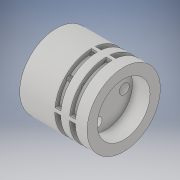
# Autodesk Inventor part: felga
Saved by Autodesk Inventor 2019 (Build 230136000, 136)
## iProperties
Created: 2019-09-09
Part Number: felga
Material: Generic
Document SubType Name: Modeling
Designer: Michal
Density: 1 g/cm^3
Appearance: Default
Author: Michal
Autodesk Inventor part; units mm, degrees
ref_plane "YZ Plane" through (0, 0, 0) normal (1, 0, 0) x (0, 1, 0)
ref_plane "XZ Plane" through (0, 0, 0) normal (0, 1, 0) x (-1, 0, 0)
ref_plane "XY Plane" through (0, 0, 0) normal (0, 0, 1) x (1, 0, 0)
sketch "Sketch1" plane through (0, 0, 0) normal (1, 0, 0) x (0, 1, 0)
  circle A0 centre (0, 0) radius 12.5
  circle A1 centre (0, 0) radius 11
  dimension "d0" = 25
  dimension "d1" = 22
  constraints: 2 centre point, 2 coincident
  measures "d0" diameter of A0
  measures "d1" diameter of A1
extrude "Extrusion1" add sketch "Sketch1" along normal blind 6.5
sketch "Sketch2" plane through (6.5, 0, 0) normal (1, 0, 0) x (0, 0, -1)
  circle A0 centre (0, 0) radius 9
  circle A1 centre (0, 0) radius 12.5
  dimension "d4" = 18
  constraints: 2 centre point, 2 coincident
  measures "d4" diameter of A0
extrude "Extrusion2" add sketch "Sketch2" along normal blind 5.5
sketch "Sketch3" plane through (12, 0, 0) normal (1, 0, 0) x (0, 0, -1)
  circle A0 centre (0, 0) radius 11
  dimension "d55" = 22
  constraints: 1 centre point, 1 coincident
  measures "d55" diameter of A0
extrude "Extrusion3" add sketch "Sketch3" along normal blind 2
sketch "Sketch4" plane through (14, 0, 0) normal (1, 0, 0) x (0, 0, -1)
  circle A0 centre (0, 0) radius 12.5
  constraints: 1 centre point, 1 coincident
extrude "Extrusion4" add sketch "Sketch4" along normal blind 3
sketch "Sketch5" plane through (17, 0, 0) normal (1, 0, 0) x (0, 0, -1)
  circle A0 centre (0, 0) radius 9
  circle A1 centre (0, 0) radius 11
  dimension "d54" = 22
  constraints: 2 centre point, 2 coincident
  measures "d54" diameter of A1
extrude "Extrusion5" add sketch "Sketch5" along normal blind 2
sketch "Sketch7" plane through (17, 0, 0) normal (1, 0, 0) x (0, 0, -1)
  line L0 (0, 0) -> (6.2, 0)
  line L1 (0, 0) -> (-3.1, 5.3694)
  line L2 (0, 0) -> (6.2, 0) construction
  line L3 (0, 0) -> (-3.1, -5.3694)
  line L4 (0, 0) -> (6.2, 0) construction
  dimension "d15" = 6.2
  dimension "d16" = 6.2
  dimension "d17" = 120
  dimension "d18" = 6.2
  dimension "d19" = 120
  constraints: 10 end point, 3 horizontal, 2 equal length
  measures "d15" distance of L0.start L0.end
  measures "d16" distance of L0.start L1.end
  measures "d17" angle of L2 L1
  measures "d18" distance of L0.start L3.end
  measures "d19" angle of L3 L4
hole "Hole1" at (17, 5.3694, 3.1) at (17, 0, -6.2) at (17, -5.3694, 3.1) direction (-1, 0, 0) diameter 3.4 end through all clearance for "Countersunk Flat Head Screw ISO 2009/7046" size "M3" standard "ISO"
sketch "Sketch8" plane through (12, 0, 0) normal (1, 0, 0) x (0, 0, -1)
  circle A0 centre (0, 0) radius 9
  circle A1 centre (0, 0) radius 9 projected
  circle A2 centre (0, 0) radius 12.5
  line L0 (-9, 0) -> (-12.5, 0)
  line L1 (-8.9507, 0.9408) -> (-12.4315, 1.3066)
  line L2 (-0.9408, -8.9507) -> (-1.3066, -12.4315)
  circle A3 centre (0, 0) radius 12.5 projected
  line L3 (0, -12.5) -> (0, -9)
  line L4 (9, 0) -> (12.5, 0)
  line L5 (0.9408, 8.9507) -> (1.3066, 12.4315)
  line L6 (0, 12.5) -> (0, 9)
  line L7 (-0.2849, 0.0299) -> (8.8591, 0.0299) construction
  line L8 (8.9507, -0.9408) -> (12.4315, -1.3066)
  constraints: 18 end point, 3 horizontal, 3 point on circle, 2 centre point, 2 vertical, 1 coincident, 1 point on line, 15 other
extrude "Extrusion7" add sketch "Sketch8" along normal blind 7 contours L4 A2 L8 A0 | A0 L6 A2 L5 | L3 A2 L2 A0 | A0 L0 A2 L1
sketch "Sketch10" plane through (17, 0, 0) normal (1, 0, 0) x (0, 0, -1)
  circle A0 centre (0, 0) radius 11
  circle A1 centre (0, 11) radius 0.75
  arc A2 (-11, 0) -> (-1.1498, -10.9397) centre (0, 0) ccw projected
  circle A3 centre (-11, 0) radius 0.75
  line L0 (0, -11) -> (0, -12.5) projected
  circle A4 centre (0, -11) radius 0.75
  circle A5 centre (11, 0) radius 0.75
  line L1 (0, 0) -> (10.9982, 0) construction
  line L2 (0, 0) -> (7.7782, 7.7782)
  line L3 (0, 0) -> (11, 0) construction
  circle A6 centre (7.7782, 7.7782) radius 0.75
  line L4 (0, 0) -> (-7.7782, 7.7782)
  line L5 (0, 0) -> (-7.7782, -7.7782)
  line L6 (0, 0) -> (7.7782, -7.7782)
  circle A7 centre (-7.7782, -7.7782) radius 0.75
  circle A8 centre (7.7782, -7.7782) radius 0.75
  circle A9 centre (-7.7782, 7.7782) radius 0.75
  dimension "d60" = 1.5
  dimension "d61" = 1.5
  dimension "d62" = 1.5
  dimension "d63" = 1.5
  dimension "d66" = 11
  dimension "d67" = 45
  dimension "d68" = 1.5
  dimension "d69" = 11
  dimension "d70" = 11
  dimension "d71" = 11
  dimension "d72" = 1.5
  dimension "d73" = 1.5
  dimension "d74" = 1.5
  constraints: 12 end point, 9 centre point, 5 coincident, 2 horizontal, 2 point on circle, 1 equal length
  measures "d60" diameter of A1
  measures "d61" diameter of A3
  measures "d62" diameter of A4
  measures "d63" diameter of A5
  measures "d66" distance of L1.start L2.end
  measures "d67" angle of L3 L2
  measures "d68" diameter of A6
  measures "d69" distance of L1.start L4.end
  measures "d70" distance of L1.start L5.end
  measures "d71" distance of L1.start L6.end
  measures "d72" diameter of A7
  measures "d73" diameter of A8
  measures "d74" diameter of A9
extrude "Extrusion8" cut sketch "Sketch10" against normal blind 7 contours A0 A5 | A0 A5 | A6 L2 A0 | A0 A6 | A8 A0 | A0 L6 A8 | L2 A6 A0 | A0 A8 L6 | A1 A0 | A0 A1 | A9 A0 L4 | L4 A0 A9 | A7 A0 L5 | L5 A0 A7 | A0 A9 | A0 A7 | A3 A0 | A0 A3
sketch "Sketch11" plane through (19, 0, 0) normal (1, 0, 0) x (0, 0, -1)
  circle A0 centre (0, 0) radius 9
  circle A1 centre (0, 0) radius 12.5
  dimension "d77" = 18
  dimension "d78" = 25
  constraints: 2 centre point, 2 coincident
  measures "d77" diameter of A0
  measures "d78" diameter of A1
extrude "Extrusion9" add sketch "Sketch11" along normal blind 4
body "Solid1"
